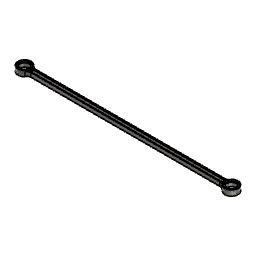
Piston Rod (Autodesk Fusion 360 design; units mm, degrees)
Autodesk Fusion 360 part; units mm, degrees
sketch "Sketch1" plane through (0, 0, 0) normal (0, 0, 1) x (1, 0, 0) in component "Component"
  circle A0 centre (0, 0) radius 1.55
  circle A1 centre (0, 0) radius 1.75
  circle A2 centre (0, 0) radius 2.25
  circle A3 centre (0, 0) radius 2.5
  circle A4 centre (77, 0) radius 1.55
  circle A5 centre (77, 0) radius 2.25
  circle A6 centre (77, 0) radius 1.75
  circle A7 centre (77, 0) radius 2.5
  line L0 (2.2913, 1) -> (74.7087, 1)
  line L1 (2.2913, -1) -> (74.7087, -1)
  arc A8 (74.3542, 0.75) -> (74.3542, -0.75) centre (77, 0) ccw
  arc A9 (2.6458, -0.75) -> (2.6458, 0.75) centre (0, 0) ccw
  line L2 (2.6458, -0.75) -> (74.3542, -0.75)
  line L3 (2.6458, 0.75) -> (74.3542, 0.75)
  line L4 (2.958, -0.5) -> (74.042, -0.5)
  arc A10 (74.042, 0.5) -> (74.042, -0.5) centre (77, 0) ccw
  line L5 (2.958, 0.5) -> (74.042, 0.5)
  arc A11 (2.958, -0.5) -> (2.958, 0.5) centre (0, 0) ccw
  point P0 (77, 0)
  dimension "d1" = 3.1
  dimension "d2" = 3.5
  dimension "d3" = 4.5
  dimension "d4" = 5
  dimension "d7" = 77
  dimension "d8" = 0
  dimension "d17" = 0.25
  constraint coincident A0.centre A1.centre
  constraint horizontal L1
  constraint coincident A3 L1.start
  constraint coincident A3 L0.start
  constraint coincident A7 L0.end
  constraint coincident A7 L1.end
  constraint concentric A7 A8
  constraint concentric A3 A9
  constraint parallel L0 L3
  constraint parallel L1 L2
  measures "d1" diameter of A0
  measures "d2" diameter of A1
  measures "d3" diameter of A2
  measures "d4" diameter of A3
extrude "Extrude1" add sketch "Sketch1" along normal mid plane 2 contours A3 | A7 makes body 1 at (2.2472, -0.1122, 0.6667) makes body 2 at (79.4876, -0.2489, -0.3333) in component "Component"
extrude "Extrude2" add sketch "Sketch1" along normal mid plane 1.5 separate body contours A1 | A6 makes body 3 at (75.7781, 1.2528, 0.5) makes body 4 at (1.7478, -0.0872, 0.5) in component "Component"
extrude "Extrude3" add sketch "Sketch1" along normal mid plane 1 contours A2 | A5 bodies 1 2 3 4 in component "Component"
extrude "Extrude4" add sketch "Sketch1" along normal mid plane 1.5 contours A3 A7 L0 L1 bodies 1 2 in component "Component"
extrude "Extrude5" add sketch "Sketch1" along normal mid plane 1.25 separate body contours L4 A10 L5 A11 makes body 5 in component "Component"
extrude "Extrude6" add sketch "Sketch1" along normal mid plane 1 contours A8 A9 L2 L3 bodies 1 5 in component "Component"
fillet "Fillet1" radius 2 4 edges at (2.2913, -1, 0) (74.7087, -1, 0) (74.7087, 1, 0) (2.2913, 1, 0) on bodies 1 in component "Component"
component "Component" placed x (1, 0, 0) y (0, 1, 0) z (0, 0, 1) at (0, 0, 0)
equation "d24 = ( 1.5 / 2 ) * 1 mm"
equation "d26 = ( 1.25 / 2 ) * 1 mm"
